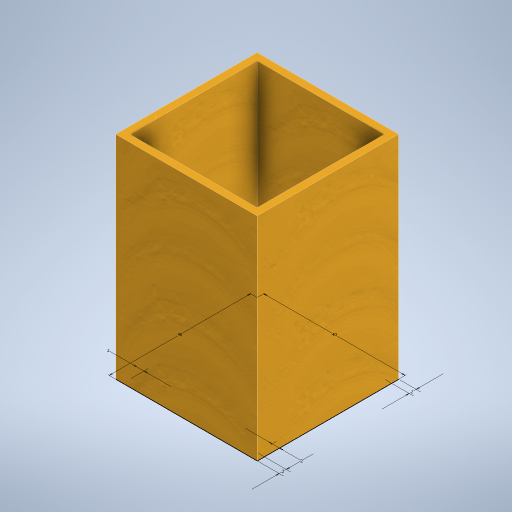
# Autodesk Inventor part: sensor_block
Saved by Autodesk Inventor 2024 (Build 280153000, 153)
## iProperties
Created: 2024-05-08
Part Number: sensor_block
Material: Brass, Soft Yellow, Welded
Document SubType Name: Modeling
Designer: kamil
Density: 8.5 g/cm^3
Appearance: Weld - Brass
Author: kamil
Autodesk Inventor part; units mm, degrees
ref_plane "YZ Plane" through (0, 0, 0) normal (1, 0, 0) x (0, 1, 0)
ref_plane "XZ Plane" through (0, 0, 0) normal (0, 1, 0) x (-1, 0, 0)
ref_plane "XY Plane" through (0, 0, 0) normal (0, 0, 1) x (1, 0, 0)
sketch "Sketch1" plane through (0, 0, 0) normal (0, 1, 0) x (-1, 0, 0)
  line L0 (0, 0) -> (40, 0)
  line L1 (40, 0) -> (40, -40)
  line L2 (40, -40) -> (0, -40)
  line L3 (0, -40) -> (0, 0)
  line L4 (2, -2) -> (38, -2)
  line L5 (38, -2) -> (38, -38)
  line L6 (38, -38) -> (2, -38)
  line L7 (2, -38) -> (2, -2)
  dimension "d0" = 40
  dimension "d1" = 40
  dimension "d2" = 2
  dimension "d3" = 2
  dimension "d4" = 2
  dimension "d5" = 2
  constraints: 16 end point, 4 parallel, 2 horizontal, 2 perpendicular
  measures "d0" distance of L1.end L2.end
  measures "d1" distance of L0.end L1.end
  measures "d2" distance between parallel lines of L4 L0
  measures "d3" distance between parallel lines of L3 L7
  measures "d4" distance between parallel lines of L1 L5
  measures "d5" distance between parallel lines of L2 L6
extrude "Extrusion1" add sketch "Sketch1" along normal blind 4 contours L4 L5 L6 L7
extrude "Extrusion2" add sketch "Sketch1" along normal blind 60
sketch "Sketch2" plane through (0, 4, 0) normal (0, 1, 0) x (1, 0, 0)
  line L0 (-26.995, 38) -> (-13.005, 38)
  line L1 (-11.1, 36.095) -> (-11.1, 18.905)
  line L2 (-13.005, 17) -> (-26.995, 17)
  line L3 (-28.9, 18.905) -> (-28.9, 36.095)
  arc A0 (-26.995, 38) -> (-28.9, 36.095) centre (-26.995, 36.095) ccw
  arc A1 (-11.1, 36.095) -> (-13.005, 38) centre (-13.005, 36.095) ccw
  arc A2 (-28.9, 18.905) -> (-26.995, 17) centre (-26.995, 18.905) ccw
  arc A3 (-13.005, 17) -> (-11.1, 18.905) centre (-13.005, 18.905) ccw
  line L4 (-38, 38) -> (-2, 38) projected
  line L5 (-38, 2) -> (-38, 38) projected
  line L6 (-30.4, 36.095) -> (-30.4, 18.905)
  arc A4 (-30.4, 18.905) -> (-26.995, 15.5) centre (-26.995, 18.905) ccw
  line L7 (-26.995, 15.5) -> (-13.005, 15.5)
  arc A5 (-13.005, 15.5) -> (-9.6, 18.905) centre (-13.005, 18.905) ccw
  line L8 (-9.6, 18.905) -> (-9.6, 36.095)
  arc A6 (-9.6, 36.095) -> (-10.1828, 38) centre (-13.005, 36.095) ccw
  arc A7 (-29.8172, 38) -> (-30.4, 36.095) centre (-26.995, 36.095) ccw
  line L9 (-29.8172, 38) -> (-10.1828, 38)
  line L10 (-40, 40) -> (-40, 0) projected
  point P0 (0, 0)
  point P1 (-11.1, 17)
  point P2 (-11.1, 38)
  point P3 (-28.9, 17)
  point P4 (-20, 38)
  point P5 (-13.005, 38)
  point P6 (-20, 17)
  dimension "d11" = 17.8
  dimension "d12" = 21
  dimension "d13" = 1.905
  dimension "d14" = 0
  dimension "d16" = 1.5
  dimension "d25" = 20
  constraints: 16 end point, 16 point on circle, 8 centre point, 8 point on line, 8 tangent, 3 equal radius, 3 parallel, 2 midpoint, 1 collinear, 1 horizontal, 1 perpendicular, 4 other
  measures "d11" distance of point (-11.1, 17) point (-28.9, 17)
  measures "d12" distance of point (-11.1, 38) point (-11.1, 17)
  measures "d13" radius of A0
  measures "d14" distance from line of L4 point (-20, 38)
  measures "d16" distance between parallel lines of L3 L6
  measures "d25" distance from line of L10 point (-20, 17)
extrude "Extrusion3" add sketch "Sketch2" along normal blind 1.2 contours A0 L3 A2 L2 A3 L1 A1 L4 A6 L8 A5 L7 A4 L6 A7
sketch "Sketch3" plane through (-38, 60, -38) normal (0, 0, 1) x (1, 0, 0)
  point P0 (38, -60)
sketch "Sketch4" plane through (0, 0, -40) normal (0, 0, -1) x (-1, 0, 0)
  line L0 (16.35, 6.9) -> (23.65, 6.9) construction
  line L1 (16.35, 4.7) -> (23.65, 4.7)
  line L2 (23.65, 9.1) -> (16.35, 9.1)
  arc A0 (16.35, 9.1) -> (16.35, 4.7) centre (16.35, 6.9) ccw
  arc A1 (23.65, 4.7) -> (23.65, 9.1) centre (23.65, 6.9) ccw
  line L3 (0, 0) -> (40, 0) projected
  line L4 (0, 0) -> (0, 60) projected
  point P0 (20, 6.9)
  dimension "d19" = 7.3
  dimension "d20" = 4.4
  dimension "d21" = 4.7
  dimension "d22" = 20
  constraints: 8 end point, 4 point on circle, 4 tangent, 2 centre point, 1 horizontal, 1 midpoint, 1 parallel
  measures "d19" distance of L0.start L0.end
  measures "d20" diameter of A1
  measures "d21" distance between parallel lines of L3 L1
  measures "d22" distance from line of L4 point (20, 6.9)
extrude "Extrusion4" cut sketch "Sketch4" against normal blind 2
body "Solid1"
